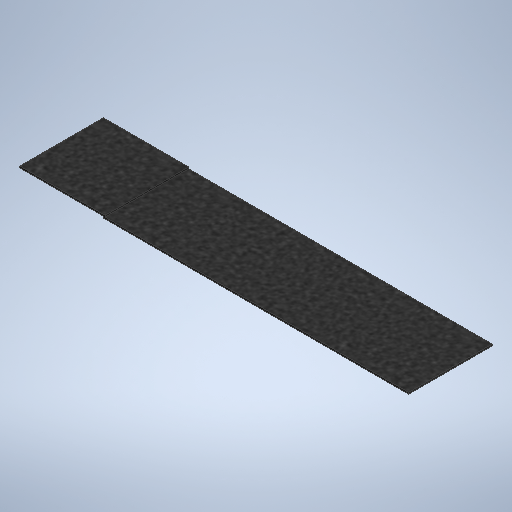
# Autodesk Inventor part: Starter_Shingle_With_Dimensions_6.5_x_30.988_Inches
Saved by Autodesk Inventor 2025 (Build 290162010, 162A)
## iProperties
Created: 2024-10-03
Part Number: Starter_Shingle_With_Dimensions_6.5_x_30.988_Inches
Material: Generic
Document SubType Name: Modeling
Designer: Tom
Density: 1 g/cm^3
Appearance: Asphalt 2
Author: Tom
Autodesk Inventor part; units mm, degrees
ref_plane "YZ Plane" through (0, 0, 0) normal (1, 0, 0) x (0, 1, 0)
ref_plane "XZ Plane" through (0, 0, 0) normal (0, 1, 0) x (-1, 0, 0)
ref_plane "XY Plane" through (0, 0, 0) normal (0, 0, 1) x (1, 0, 0)
sketch "Sketch1" plane through (0, 0, 0) normal (0, 0, 1) x (1, 0, 0)
  line L0 (0, 0) -> (602.9452, 0)
  line L1 (602.9452, 0) -> (602.9452, 3.175)
  line L2 (602.9452, 3.175) -> (3.175, 3.175)
  line L3 (3.175, 3.175) -> (3.175, 6.35)
  line L4 (3.175, 6.35) -> (-165.1, 6.35)
  line L5 (-165.1, 6.35) -> (-165.1, 3.175)
  line L6 (-165.1, 3.175) -> (0, 3.175)
  line L7 (0, 3.175) -> (0, 0)
  dimension "d0" = 165.1
  dimension "d1" = 3.175
  dimension "d2" = 3.175
  dimension "d3" = 3.175
  dimension "d4" = 3.175
  dimension "d10" = 602.9452
  constraints: 16 end point, 6 perpendicular, 1 horizontal, 1 point on line
  measures "d0" distance of L5.end L6.end
  measures "d1" distance between parallel lines of L4 L6
  measures "d2" distance between parallel lines of L3 L7
  measures "d3" distance between parallel lines of L2 L0
  measures "d4" distance of L6.end L0.start
  measures "d10" distance from line of L1.end L7
extrude "Extrusion2" add sketch "Sketch1" along normal blind 165.1
body "Solid2"
